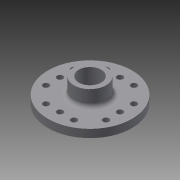
# Autodesk Inventor part: horn
Saved by Autodesk Inventor 2015 (Build 190159000, 159)
## iProperties
Created: 2015-06-27
Part Number: horn
Material: Genérico
Document SubType Name: Modeling
Designer: Roberto
Density: 1 g/cm^3
Appearance: Valor por defecto
Author: Roberto
Autodesk Inventor part; units mm, degrees
ref_plane "YZ Plane" through (0, 0, 0) normal (1, 0, 0) x (0, 1, 0)
ref_plane "XZ Plane" through (0, 0, 0) normal (0, 1, 0) x (-1, 0, 0)
ref_plane "XY Plane" through (0, 0, 0) normal (0, 0, 1) x (1, 0, 0)
sketch "Boceto1" plane through (0, 0, 0) normal (0, 0, 1) x (1, 0, 0)
  circle A0 centre (0, 0) radius 10.5
  dimension "d0" = 21
  constraints: 1 centre point, 1 coincident
  measures "d0" diameter of A0
extrude "Extrusión1" add sketch "Boceto1" along normal blind 2
sketch "Boceto2" plane through (0, 0, 2) normal (0, 0, 1) x (1, 0, 0)
  circle A0 centre (0, 0) radius 4
  dimension "d4" = 8
  constraints: 1 centre point, 1 coincident
  measures "d4" diameter of A0
extrude "Extrusión2" add sketch "Boceto2" along normal blind 4
fillet "Empalme1" radius 1 1 edges at (-4, 0, 2)
sketch "Boceto3" plane through (0, 0, 6) normal (0, 0, 1) x (1, 0, 0)
  circle A0 centre (0, 0) radius 4 projected
  circle A1 centre (0, 0) radius 2.8
  dimension "d8" = 5.6
  constraints: 1 centre point, 1 coincident
  measures "d8" diameter of A1
extrude "Extrusión3" cut sketch "Boceto3" against normal blind 4 contours A1
sketch "Boceto4" plane through (0, 0, 2) normal (0, 0, 1) x (1, 0, 0)
  circle A0 centre (0, 0) radius 1.475
  dimension "d11" = 2.95
  constraints: 1 centre point, 1 coincident
  measures "d11" diameter of A0
extrude "Extrusión4" cut sketch "Boceto4" against normal up to surface (2 mm away)
sketch "Boceto5" plane through (0, 0, 0) normal (0, 0, -1) x (-1, 0, 0)
  circle A0 centre (0, 0) radius 1.475 projected
  circle A1 centre (0, 0) radius 3
  dimension "d14" = 6
  constraints: 1 centre point, 1 coincident
  measures "d14" diameter of A1
extrude "Extrusión5" cut sketch "Boceto5" against normal blind 0.5
sketch "Boceto6" plane through (0, 0, 0) normal (0, 0, -1) x (-1, 0, 0)
  line L0 (11.1976, -7.5) -> (-9.8806, -7.5)
  circle A0 centre (0, -7.5) radius 0.75
  circle A1 centre (3.5, -7.5) radius 0.75
  circle A2 centre (-3.5, -7.5) radius 0.75
  circle A3 centre (7.5, 0) radius 0.75
  circle A4 centre (7.5, 3.5) radius 0.75
  circle A5 centre (7.5, -3.5) radius 0.75
  circle A6 centre (0, 7.5) radius 0.75
  circle A7 centre (-3.5, 7.5) radius 0.75
  circle A8 centre (3.5, 7.5) radius 0.75
  circle A9 centre (-7.5, 0) radius 0.75
  circle A10 centre (-7.5, -3.5) radius 0.75
  circle A11 centre (-7.5, 3.5) radius 0.75
  point P0 (0, 0)
  dimension "d17" = 7.5
  dimension "d18" = 1.5
  dimension "d19" = 3.5
  dimension "d20" = 3.5
  dimension "d23" = 360
  constraints: 12 centre point, 3 point on line, 2 end point, 2 equal radius, 1 horizontal, 25 other
  measures "d17" distance from line of point (0, 0) L0
  measures "d18" diameter of A0
  measures "d19" distance of A0.centre A1.centre
  measures "d20" distance of A2.centre A0.centre
extrude "Extrusión6" cut sketch "Boceto6" against normal through all
